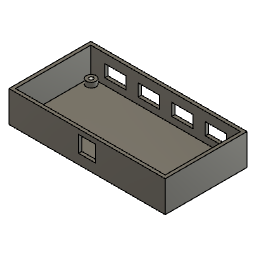
USB Power Box v5 (Autodesk Fusion 360 design; units mm, degrees)
Autodesk Fusion 360 part; units mm, degrees
note: some values were not read from the file. Set by a fixed rule: which sketch regions a step uses.
sketch "Sketch1" plane through (0, 0, 0) normal (0, 1, 0) x (1, 0, 0)
  line L0 (0, 0) -> (95.5, 0)
  line L1 (95.5, 0) -> (95.5, 50)
  line L2 (95.5, 50) -> (0, 50)
  line L3 (0, 50) -> (0, 0)
  dimension "d1" = 95.5
  dimension "d2" = 50
  constraint horizontal L0
  constraint vertical L1
  constraint horizontal L2
  constraint vertical L3
  constraint coincident L0.start L3.end
  measures "d1" distance of L0.start L0.end
  measures "d2" distance of L0.start L2.end
extrude "Extrude1" add sketch "Sketch1" along normal blind 19
sketch "Sketch6" plane through (0, 19, 0) normal (0, 1, 0) x (-1, 0, 0)
  line L0 (0, -50) -> (0, 0)
  line L1 (0, 0) -> (-95.5, 0)
  line L2 (-95.5, 0) -> (-95.5, -50)
  line L3 (-95.5, -50) -> (0, -50)
  line L4 (-2, -2) -> (-93.5, -2)
  line L5 (-93.5, -2) -> (-93.5, -48)
  line L6 (-93.5, -48) -> (-2, -48)
  line L7 (-2, -48) -> (-2, -2)
  dimension "d39" = 91.5
  dimension "d40" = 46
  constraint horizontal L4
  constraint vertical L5
  constraint horizontal L6
  constraint vertical L7
  measures "d39" distance of L4.start L4.end
  measures "d40" distance of L4.start L6.end
extrude "Extrude5" cut sketch "Sketch6" against normal blind 17 contours L4 L5 L6 L7
sketch "Sketch8" plane through (0, 0, 0) normal (0, 0, 1) x (1, 0, 0)
  line L0 (0, 0) -> (95.5, 0)
  line L1 (95.5, 0) -> (95.5, 19)
  line L2 (95.5, 19) -> (0, 19)
  line L3 (0, 19) -> (0, 0)
  line L4 (0, 19) -> (42.5, 19)
  line L5 (42.5, 19) -> (42.5, 6)
  line L6 (42.5, 6) -> (0, 6)
  line L7 (0, 6) -> (0, 19)
  line L8 (42.5, 6) -> (52.9, 6)
  line L9 (52.9, 6) -> (52.9, 16)
  line L10 (52.9, 16) -> (42.5, 16)
  line L11 (42.5, 16) -> (42.5, 6)
  dimension "d66" = 42.5
  dimension "d67" = 13
  dimension "d68" = 10.4
  dimension "d69" = 10
  constraint horizontal L4
  constraint vertical L5
  constraint horizontal L6
  constraint vertical L7
  constraint coincident L2.end L3.start
  constraint horizontal L8
  constraint vertical L9
  constraint horizontal L10
  constraint vertical L11
  measures "d66" distance of L2.end L4.end
  measures "d67" distance of L2.end L6.end
  measures "d68" distance of L5.end L8.end
  measures "d69" distance of L5.end L10.end
extrude "Extrude7" cut sketch "Sketch8" against normal blind 2 contours L5 L8 L9 L10 L11
sketch "Sketch9" plane through (0, 0, -50) normal (0, 0, -1) x (-1, 0, 0)
  line L0 (-95.5, 0) -> (0, 0)
  line L1 (0, 0) -> (0, 19)
  line L2 (0, 19) -> (-95.5, 19)
  line L3 (-95.5, 19) -> (-95.5, 0)
  line L4 (-95.5, 19) -> (-51.5, 19)
  line L5 (-51.5, 19) -> (-51.5, 6)
  line L6 (-51.5, 6) -> (-95.5, 6)
  line L7 (-95.5, 6) -> (-95.5, 19)
  line L8 (-51.5, 6) -> (-64.5, 6)
  line L9 (-64.5, 6) -> (-64.5, 13.5)
  line L10 (-64.5, 13.5) -> (-51.5, 13.5)
  line L11 (-51.5, 13.5) -> (-51.5, 6)
  line L12 (-64.5, 6) -> (-72, 6)
  line L13 (-72, 6) -> (-72, 13.5)
  line L14 (-72, 13.5) -> (-64.5, 13.5)
  line L15 (-64.5, 13.5) -> (-64.5, 6)
  line L16 (-72, 6) -> (-85, 6)
  line L17 (-85, 6) -> (-85, 13.5)
  line L18 (-85, 13.5) -> (-72, 13.5)
  line L19 (-72, 13.5) -> (-72, 6)
  line L20 (-51.5, 6) -> (-44, 6)
  line L21 (-44, 6) -> (-44, 13.5)
  line L22 (-44, 13.5) -> (-51.5, 13.5)
  line L23 (-51.5, 13.5) -> (-51.5, 6)
  line L24 (-44, 6) -> (-31, 6)
  line L25 (-31, 6) -> (-31, 13.5)
  line L26 (-31, 13.5) -> (-44, 13.5)
  line L27 (-44, 13.5) -> (-44, 6)
  line L28 (-31, 6) -> (-23.5, 6)
  line L29 (-23.5, 6) -> (-23.5, 13.5)
  line L30 (-23.5, 13.5) -> (-31, 13.5)
  line L31 (-31, 13.5) -> (-31, 6)
  line L32 (-23.5, 6) -> (-10.5, 6)
  line L33 (-10.5, 6) -> (-10.5, 13.5)
  line L34 (-10.5, 13.5) -> (-23.5, 13.5)
  line L35 (-23.5, 13.5) -> (-23.5, 6)
  dimension "d72" = 44
  dimension "d73" = 13
  dimension "d74" = 13
  dimension "d75" = 7.5
  dimension "d76" = 7.5
  dimension "d77" = 7.5
  dimension "d78" = 13
  dimension "d79" = 7.5
  dimension "d80" = 7.5
  dimension "d81" = 7.5
  dimension "d82" = 13
  dimension "d83" = 7.5
  dimension "d84" = 7.5
  dimension "d85" = 7.5
  dimension "d86" = 13
  dimension "d87" = 7.5
  constraint horizontal L4
  constraint vertical L5
  constraint horizontal L6
  constraint vertical L7
  constraint coincident L2.end L3.start
  constraint horizontal L8
  constraint vertical L9
  constraint horizontal L10
  constraint vertical L11
  constraint horizontal L12
  constraint vertical L13
  constraint horizontal L14
  constraint vertical L15
  constraint horizontal L16
  constraint vertical L17
  constraint horizontal L18
  constraint vertical L19
  constraint horizontal L20
  constraint vertical L21
  constraint horizontal L22
  constraint vertical L23
  constraint horizontal L24
  constraint vertical L25
  constraint horizontal L26
  constraint vertical L27
  constraint horizontal L28
  constraint vertical L29
  constraint horizontal L30
  constraint vertical L31
  constraint horizontal L32
  constraint vertical L33
  constraint horizontal L34
  constraint vertical L35
  measures "d72" distance of L2.end L4.end
  measures "d73" distance of L2.end L6.end
  measures "d74" distance of L5.end L8.end
  measures "d75" distance of L5.end L10.end
  measures "d76" distance of L8.end L12.end
  measures "d77" distance of L8.end L9.end
  measures "d78" distance of L12.end L16.end
  measures "d79" distance of L12.end L13.end
  measures "d80" distance of L5.end L20.end
  measures "d81" distance of L5.end L10.end
  measures "d82" distance of L20.end L24.end
  measures "d83" distance of L20.end L21.end
  measures "d84" distance of L24.end L28.end
  measures "d85" distance of L24.end L25.end
  measures "d86" distance of L28.end L32.end
  measures "d87" distance of L28.end L29.end
extrude "Extrude8" cut sketch "Sketch9" against normal blind 2 contours L6 L13 L16 L17 L18 L19 | L5 L6 L8 L9 L10 L11 L15 L23 | L21 L24 L25 L26 L27 L31 | L29 L32 L33 L34 L35
sketch "Sketch10" plane through (0, 0, 0) normal (0, 1, 0) x (1, 0, 0)
  line L0 (2, 2) -> (5.75, 2)
  line L1 (5.75, 2) -> (5.75, 5.5)
  line L2 (5.75, 5.5) -> (2, 5.5)
  line L3 (2, 5.5) -> (2, 2)
  circle A0 centre (5.75, 5.5) radius 3
  line L4 (2, 48) -> (5.75, 48)
  line L5 (5.75, 48) -> (5.75, 44.5)
  line L6 (5.75, 44.5) -> (2, 44.5)
  line L7 (2, 44.5) -> (2, 48)
  circle A1 centre (5.75, 44.5) radius 3
  line L8 (93.5, 48) -> (89.75, 48)
  line L9 (89.75, 48) -> (89.75, 44.5)
  line L10 (89.75, 44.5) -> (93.5, 44.5)
  line L11 (93.5, 44.5) -> (93.5, 48)
  circle A2 centre (89.75, 44.5) radius 3
  line L12 (93.5, 2) -> (89.75, 2)
  line L13 (89.75, 2) -> (89.75, 5.5)
  line L14 (89.75, 5.5) -> (93.5, 5.5)
  line L15 (93.5, 5.5) -> (93.5, 2)
  circle A3 centre (89.75, 5.5) radius 3
  dimension "d93" = 3.75
  dimension "d94" = 3.5
  dimension "d95" = 6
  dimension "d96" = 3.75
  dimension "d97" = 3.5
  dimension "d98" = 6
  dimension "d99" = 3.75
  dimension "d100" = 3.5
  dimension "d101" = 6
  dimension "d102" = 3.75
  dimension "d103" = 3.5
  dimension "d104" = 6
  constraint horizontal L0
  constraint vertical L1
  constraint horizontal L2
  constraint vertical L3
  constraint coincident L1.end L2.start
  constraint horizontal L4
  constraint vertical L5
  constraint horizontal L6
  constraint vertical L7
  constraint coincident L5.end L6.start
  constraint horizontal L8
  constraint vertical L9
  constraint horizontal L10
  constraint vertical L11
  constraint coincident L9.end L10.start
  constraint horizontal L12
  constraint vertical L13
  constraint horizontal L14
  constraint vertical L15
  constraint coincident L13.end L14.start
  measures "d93" distance of L0.start L0.end
  measures "d94" distance of L0.start L2.end
  measures "d95" diameter of A0
  measures "d96" distance of L4.start L4.end
  measures "d97" distance of L4.start L6.end
  measures "d98" diameter of A1
  measures "d99" distance of L8.start L8.end
  measures "d100" distance of L8.start L10.end
  measures "d101" diameter of A2
  measures "d102" distance of L12.start L12.end
  measures "d103" distance of L12.start L14.end
  measures "d104" diameter of A3
extrude "Extrude9" add sketch "Sketch10" along normal blind 5 contours L1 L2 A0 | L1 L2 A0 | L5 L6 A1 | L5 L6 A1 | L9 L10 A2 | L9 L10 A2 | L13 L14 A3 | L13 L14 A3
hole "Hole5" at (5.75, 5, -44.5) direction (0, -1, 0) diameter 2.529 depth 5 tip angle 180
thread "Thread5" "ISO Metric profile 3.0 M3x0.5 6H"
hole "Hole6" at (89.75, 5, -44.5) direction (0, -1, 0) diameter 2.529 depth 5 tip angle 180
thread "Thread6" "ISO Metric profile 3.0 M3x0.5 6H"
hole "Hole7" at (89.75, 5, -5.5) direction (0, -1, 0) diameter 2.529 depth 5 tip angle 180
thread "Thread7" "ISO Metric profile 3.0 M3x0.5 6H"
hole "Hole8" at (5.75, 5, -5.5) direction (0, -1, 0) diameter 2.529 depth 5 tip angle 180
thread "Thread8" "ISO Metric profile 3.0 M3x0.5 6H"
